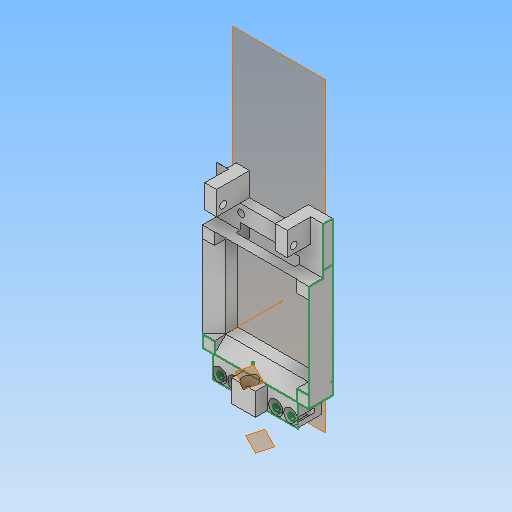
# Autodesk Inventor part: 09_Opentrons_Autofocus_LED_Module
Saved by Autodesk Inventor 2019.4 (Build 234330000, 330)
## iProperties
Created: 2020-11-27
Part Number: 09_Opentrons_Autofocus_LED_Module
Material: Generic
Document SubType Name: Modeling
Designer: diederichbenedict
Density: 1 g/cm^3
Appearance: Default
Author: diederichbenedict
Autodesk Inventor part; units mm, degrees
ref_plane "YZ Plane" through (0, 0, 0) normal (1, 0, 0) x (0, 1, 0)
ref_plane "XZ Plane" through (0, 0, 0) normal (0, 1, 0) x (-1, 0, 0)
ref_plane "XY Plane" through (0, 0, 0) normal (0, 0, 1) x (1, 0, 0)
ref_plane "Work Plane1" through (0, 0, 0) normal (0, 0, 1) x (1, 0, 0)
sketch "Sketch1" plane through (0, 0, 0) normal (0, 0, 1) x (1, 0, 0)
  circle A0 centre (8.8475, 49.7489) radius 1.45 construction
  circle A1 centre (9.593, -3.6603) radius 1.45 construction
  circle A2 centre (-7.7223, -3.6603) radius 1.45 construction
  circle A3 centre (-14.1116, -11.6603) radius 1.45 construction
  circle A4 centre (-7.7223, -11.6603) radius 1.45 construction
  circle A5 centre (9.593, -11.6603) radius 1.45 construction
  circle A6 centre (15.9823, -11.6603) radius 1.45 construction
  circle A7 centre (-6.9768, 49.7489) radius 1.45 construction
  line L0 (-17.1585, 69.3865) -> (-2.1585, 69.3865) construction
  line L1 (-2.1585, 69.3865) -> (-2.1585, 62.7008) construction
  line L2 (-2.1585, 62.7008) -> (-2.1585, 59.9787) construction
  line L3 (-2.1585, 59.9787) -> (-2.1585, 53.293) construction
  line L4 (-2.1585, 53.293) -> (-17.1585, 53.293) construction
  line L5 (-17.1585, 53.293) -> (-17.1585, -14.6603) construction
  line L6 (-17.1585, -14.6603) -> (18.8415, -14.6603) construction
  line L7 (18.8415, -14.6603) -> (18.8415, 91.3397) construction
  line L8 (-6.8647, 91.3397) -> (18.8415, 91.3397) construction
  line L9 (-6.8647, 103.3397) -> (-6.8647, 91.3397) construction
  line L10 (-17.1585, 103.3397) -> (-6.8647, 103.3397) construction
  line L11 (-17.1585, 69.3865) -> (-17.1585, 103.3397) construction
  line L12 (18.4353, 34.7801) -> (-16.5647, 34.7801)
  line L13 (-16.5647, 34.7801) -> (-16.5647, -0.2199)
  line L14 (-16.5647, -0.2199) -> (18.4353, -0.2199)
  line L15 (18.4353, -0.2199) -> (18.4353, 34.7801)
  line L16 (18.4353, 34.7801) -> (-16.5647, -0.2199) construction
  line L17 (-16.5647, 34.7801) -> (18.4353, -0.2199) construction
  line L18 (23.4353, -5.2199) -> (-21.5647, -5.2199)
  line L19 (-21.5647, -5.2199) -> (-21.5647, 39.7801)
  line L20 (-21.5647, 39.7801) -> (23.4353, 39.7801)
  line L21 (23.4353, 39.7801) -> (23.4353, -5.2199)
  line L22 (23.4353, -5.2199) -> (-21.5647, 39.7801) construction
  line L23 (-21.5647, -5.2199) -> (23.4353, 39.7801) construction
  line L24 (-17.1585, -14.6603) -> (18.8415, -14.6603)
  line L25 (18.8415, -14.6603) -> (18.8415, -5.2199)
  line L26 (18.8415, -5.2199) -> (-17.1585, -5.2199)
  line L27 (-17.1585, -5.2199) -> (-17.1585, -14.6603)
  circle A8 centre (-14.1116, -11.6603) radius 1.45
  circle A9 centre (-7.7223, -11.6603) radius 1.45
  circle A10 centre (9.593, -11.6603) radius 1.45
  circle A11 centre (15.9823, -11.6603) radius 1.45
  line L28 (15.9353, 32.2801) -> (15.9353, 2.2801) projected
  line L29 (15.9353, 2.2801) -> (-14.0647, 2.2801) projected
  line L30 (-14.0647, 2.2801) -> (-14.0647, 32.2801) projected
  line L31 (-14.0647, 32.2801) -> (15.9353, 32.2801) projected
  point P0 (0, 0)
  point P1 (0.9353, 17.2801)
  dimension "d0" = 35
  dimension "d1" = 35
  dimension "d2" = 45
  dimension "d3" = 45
  constraints: 32 end point, 6 parallel, 4 centre point, 4 coincident, 4 concentric, 4 midpoint, 3 horizontal, 3 perpendicular, 2 point on line
  measures "d0" distance of L14.end L13.end
  measures "d1" distance of L13.end L12.end
  measures "d2" distance of L19.end L20.end
  measures "d3" distance of L18.end L19.end
extrude "Extrusion1" add sketch "Sketch1" along normal blind 10 contours L18 L19 L20 L21 | L25 L24 L27 L18
sketch "Sketch2" plane through (-16.5647, 34.7801, 0) normal (0, -1, 0) x (1, 0, 0)
  line L0 (0, 0) -> (0, 10) projected
  line L1 (35, 0) -> (0, 0) projected
  line L2 (35, 0) -> (35, 10) projected
  line L3 (0, 10) -> (35, 10) projected
  line L4 (0, 0) -> (0, 10) projected
  line L5 (5, 0) -> (-5, 10)
  line L6 (5, 0) -> (19.1421, 0) construction
  line L7 (-5, 10) -> (5, 10)
  line L8 (40, 10) -> (-5, 10) projected
  line L9 (5, 0) -> (5, 10)
  line L10 (-5, 0) -> (-5, 10) projected
  line L11 (12.5, -7.6051) -> (12.5, -58.2325)
  line L12 (40, 10) -> (30, 0)
  line L13 (40, 0) -> (-5, 0) projected
  line L14 (40, 10) -> (54.1421, 10) construction
  line L15 (30, 0) -> (40, 10)
  line L16 (30, 0) -> (30, 10)
  line L17 (30, 0) -> (40, 0) construction
  line L18 (30, 10) -> (40, 10)
  point P0 (16.5647, 0)
  dimension "d6" = 135
  dimension "d7" = 10
  dimension "d9" = 45
  dimension "d10" = 0
  dimension "d11" = 135
  dimension "d12" = 90
  constraints: 22 end point, 3 equal length, 3 horizontal, 2 point on line, 1 collinear, 1 perpendicular, 1 vertical, 4 other
  measures "d6" angle of L6 L5
  measures "d7" distance of L7.end L5.start
  measures "d9" angle of L7 L5
  measures "d10" distance from line of L10 L5.end
  measures "d11" angle of L12 L14
  measures "d12" angle of L17 L16
extrude "Extrusion2" cut sketch "Sketch2" along normal up to surface (35 mm away) contours L5 L7 L0 | L0 L3 L9 L5 | L9 L3 L16 L1 | L16 L3 L2 L12 | L2 L8 L12
sketch "Sketch3" plane through (0, 0, 10) normal (0, 0, 1) x (1, 0, 0)
  line L0 (23.4353, -0.2199) -> (-21.5647, -0.2199) projected
  line L1 (-21.5647, -0.2199) -> (-21.5647, -5.2199) projected
  line L2 (-21.5647, -5.2199) -> (-17.1585, -5.2199) projected
  line L3 (-17.1585, -5.2199) -> (-17.1585, -14.6603) projected
  line L4 (-17.1585, -14.6603) -> (18.8415, -14.6603) projected
  line L5 (18.8415, -14.6603) -> (18.8415, -5.2199) projected
  line L6 (18.8415, -5.2199) -> (23.4353, -5.2199) projected
  line L7 (23.4353, -5.2199) -> (23.4353, -0.2199) projected
  circle A0 centre (15.9823, -11.6603) radius 1.45 projected
  circle A1 centre (9.593, -11.6603) radius 1.45 projected
  circle A2 centre (-7.7223, -11.6603) radius 1.45 projected
  circle A3 centre (-14.1116, -11.6603) radius 1.45 projected
  circle A4 centre (0.9353, 17.3993) radius 10.125 projected
  point P0 (0, 0)
ref_plane "Work Plane2" through (0.9353, 17.3993, 8.4308) normal (0, 0, 1) x (1, 0, 0)
pattern_circular "Circular Pattern1" count 2 over 90 about axis through (0.9353, 17.3993, 10) along (0, 0, 1) of "Extrusion2"
sketch "Sketch4" plane through (0, 0, 10) normal (0, 0, 1) x (1, 0, 0)
  line L0 (-16.4454, -5.1007) -> (-16.4454, -0.2199) projected
  line L1 (-16.4454, -0.2199) -> (-21.5647, -0.2199) projected
  line L2 (-21.5647, -0.2199) -> (-21.5647, -5.2199) projected
  line L3 (-21.5647, -5.2199) -> (-17.1585, -5.2199) projected
  line L4 (-17.1585, -5.2199) -> (-17.1585, -14.6603) projected
  line L5 (-17.1585, -14.6603) -> (18.8415, -14.6603) projected
  line L6 (18.8415, -14.6603) -> (18.8415, -5.2199) projected
  line L7 (18.8415, -5.2199) -> (23.4353, -5.2199) projected
  line L8 (23.4353, -5.2199) -> (23.4353, -0.2199) projected
  line L9 (23.4353, -0.2199) -> (18.5546, -0.2199) projected
  line L10 (18.5546, -0.2199) -> (18.5546, -5.1007) projected
  line L11 (18.5546, -5.1007) -> (-16.4454, -5.1007) projected
  circle A0 centre (15.9823, -11.6603) radius 1.45 projected
  circle A1 centre (9.593, -11.6603) radius 1.45 projected
  circle A2 centre (-7.7223, -11.6603) radius 1.45 projected
  circle A3 centre (-14.1116, -11.6603) radius 1.45 projected
  point P0 (0, 0)
hole "Hole1" at (-14.1116, -11.6603, 10) at (-7.7223, -11.6603, 10) at (9.593, -11.6603, 10) at (15.9823, -11.6603, 10) direction (0, 0, -1) diameter 2.9 end through all counterbore diameter 6 counterbore depth 7
sketch "Sketch5" plane through (0, 0, 10) normal (0, 0, 1) x (1, 0, 0)
  line L0 (-2.5647, -10.9312) -> (-2.5647, -13.1962)
  line L1 (4.4353, -10.9312) -> (4.4353, -13.1962)
  line L2 (-7.7223, -14.6603) -> (9.593, -14.6603) projected
  line L3 (18.5546, -5.1007) -> (-16.4454, -5.1007) projected
  line L4 (5.9353, -5.1007) -> (-4.0647, -5.1007)
  line L5 (-4.0647, -5.1007) -> (-4.0647, -14.6603)
  line L6 (-4.0647, -14.6603) -> (5.9353, -14.6603)
  line L7 (5.9353, -14.6603) -> (5.9353, -5.1007)
  line L8 (5.9353, -5.1007) -> (-4.0647, -14.6603) construction
  line L9 (-4.0647, -5.1007) -> (5.9353, -14.6603) construction
  point P0 (0, 0)
  point P1 (0.9353, -9.8805)
  dimension "d25" = 0
  dimension "d26" = 10
  constraints: 16 end point, 2 midpoint, 2 parallel, 2 vertical, 1 horizontal, 1 perpendicular, 1 point on line, 4 other
  measures "d25" distance between parallel lines of L3 L4
  measures "d26" distance between parallel lines of L7 L5
extrude "Extrusion3" add sketch "Sketch5" along normal blind 5
ref_plane "Work Plane3" through (3.4683, -3.8016, 13.7177) normal (0, 0.9848078, 0.173648) x (0.426172, 0.1570893, -0.8908986)
sketch "Sketch6" plane through (3.4683, -3.8016, 13.7177) normal (0, 0.9848078, 0.173648) x (0.426172, 0.1570893, -0.8908986)
  circle A0 centre (0, 2.8) radius 3 projected
  circle A1 centre (0, 2.8) radius 3
  point P0 (11.3402, 9.1762)
  dimension "d29" = 6
  constraints: 1 centre point, 1 coincident
  measures "d29" diameter of A1
extrude "Extrusion4" cut sketch "Sketch6" against normal through all
ref_plane "Work Plane4" through (3.4683, -29.6528, 9.1595) normal (0, 0.9848078, 0.173648) x (0.426172, 0.1570893, -0.8908986)
sketch "Sketch7" plane through (3.4683, -29.6528, 9.1595) normal (0, 0.9848078, 0.173648) x (0.426172, 0.1570893, -0.8908986)
  circle A0 centre (0, 2.8) radius 3.5 projected
  circle A1 centre (0, 2.8) radius 4
  point P0 (11.3402, 9.1762)
  dimension "d33" = 8
  constraints: 1 centre point, 1 coincident
  measures "d33" diameter of A1
ref_plane "Work Plane5" through (-3.7225, -12.4362, 6.5391) normal (0, -0.9848078, -0.173648) x (0.9046422, -0.0740039, 0.4196975)
extrude "Extrusion5" cut sketch "Sketch7" along normal up to surface (16.5 mm away) contours A0 | A1
sketch "Sketch8" plane through (-21.5647, 39.7801, 0) normal (0, 1, 0) x (1, 0, 0)
  line L0 (5.1193, -10) -> (5.1193, -9.8807) projected
  line L1 (5.1193, -9.8807) -> (40.1193, -9.8807) projected
  line L2 (40.1193, -9.8807) -> (40.1193, -10) projected
  line L3 (45, -10) -> (40.1193, -10) projected
  line L4 (45, 0) -> (45, -10) projected
  line L5 (45, 0) -> (0, 0) projected
  line L6 (0, 0) -> (0, -10) projected
  line L7 (5.1193, -10) -> (0, -10) projected
  line L8 (30.575, -5.7143) -> (27, -5.7143) projected
  line L9 (30.575, -5.7143) -> (30.575, -4.7143) projected
  line L10 (27, -4.7143) -> (30.575, -4.7143) projected
  line L11 (18, -4.7143) -> (27, -4.7143) projected
  line L12 (14.425, -4.7143) -> (18, -4.7143) projected
  line L13 (14.425, -5.7143) -> (14.425, -4.7143) projected
  line L14 (18, -5.7143) -> (14.425, -5.7143) projected
  line L15 (27, -5.7143) -> (18, -5.7143) projected
  line L16 (5, 0) -> (40, 0) projected
  line L17 (35, -5.7143) -> (10, -5.7143)
  line L18 (10, -5.7143) -> (10, 0)
  line L19 (10, 0) -> (35, 0)
  line L20 (35, 0) -> (35, -5.7143)
  point P0 (21.5647, 0)
  dimension "d36" = 10
  dimension "d37" = 10
  constraints: 8 end point, 2 parallel, 1 horizontal, 1 perpendicular, 1 point on line
  measures "d36" distance between parallel lines of L20 L4
  measures "d37" distance between parallel lines of L6 L18
extrude "Extrusion6" cut sketch "Sketch8" against normal up to surface (5 mm away) contours L5 L20 L17 L9 L10 L11 L12 L13 L18 | L13 L12 L11 L10 L9 L8 L15 L14
sketch "Sketch9" plane through (0, 0, 0) normal (0, 0, -1) x (-1, 0, 0)
  line L0 (-13.4353, 34.7801) -> (-13.4353, 39.7801) projected
  line L1 (-23.4353, 39.7801) -> (-13.4353, 39.7801) projected
  line L2 (-23.4353, -5.2199) -> (-23.4353, 39.7801) projected
  line L3 (-18.8415, -5.2199) -> (-23.4353, -5.2199) projected
  line L4 (-18.8415, -14.6603) -> (-18.8415, -5.2199) projected
  line L5 (17.1585, -14.6603) -> (-18.8415, -14.6603) projected
  line L6 (17.1585, -5.2199) -> (17.1585, -14.6603) projected
  line L7 (21.5647, -5.2199) -> (17.1585, -5.2199) projected
  line L8 (21.5647, 39.7801) -> (21.5647, -5.2199) projected
  line L9 (11.5647, 39.7801) -> (21.5647, 39.7801) projected
  line L10 (11.5647, 39.7801) -> (11.5647, 34.7801) projected
  line L11 (11.5647, 34.7801) -> (16.5647, 34.7801) projected
  line L12 (16.5647, 34.7801) -> (16.5647, -0.2199) projected
  line L13 (16.5647, -0.2199) -> (-18.4353, -0.2199) projected
  line L14 (-18.4353, -0.2199) -> (-18.4353, 4.8993) projected
  line L15 (-18.4353, 4.8993) -> (-18.5546, 4.8993) projected
  line L16 (-18.5546, 4.8993) -> (-18.5546, 29.8993) projected
  line L17 (-18.5546, 29.8993) -> (-18.4353, 29.8993) projected
  line L18 (-18.4353, 29.8993) -> (-18.4353, 34.7801) projected
  line L19 (-18.4353, 34.7801) -> (-13.4353, 34.7801) projected
  circle A0 centre (14.1116, -11.6603) radius 1.45 projected
  circle A1 centre (7.7223, -11.6603) radius 1.45 projected
  circle A2 centre (-9.593, -11.6603) radius 1.45 projected
  circle A3 centre (-15.9823, -11.6603) radius 1.45 projected
  line L20 (-8.9353, 55.6182) -> (7.0647, 55.6182) projected
  line L21 (7.0647, 55.6182) -> (7.0647, 61.2182) projected
  line L22 (7.0647, 61.2182) -> (-8.9353, 61.2182) projected
  line L23 (-8.9353, 61.2182) -> (-8.9353, 55.6182) projected
  circle A4 centre (7.6659, 72.0993) radius 0.5 projected
  circle A5 centre (-9.7637, 72.0993) radius 0.5 projected
  line L24 (3.5647, 69.0382) -> (3.5647, 73.4382) projected
  line L25 (3.5647, 73.4382) -> (7.1397, 73.4382) projected
  arc A6 (9.1397, 71.4382) -> (7.1397, 73.4382) centre (7.1397, 71.4382) ccw projected
  line L26 (9.1397, 71.4382) -> (9.1397, 32.1382) projected
  arc A7 (7.1397, 30.1382) -> (9.1397, 32.1382) centre (7.1397, 32.1382) ccw projected
  line L27 (7.1397, 30.1382) -> (-9.0103, 30.1382) projected
  arc A8 (-11.0103, 32.1382) -> (-9.0103, 30.1382) centre (-9.0103, 32.1382) ccw projected
  line L28 (-11.0103, 32.1382) -> (-11.0103, 71.4382) projected
  arc A9 (-9.0103, 73.4382) -> (-11.0103, 71.4382) centre (-9.0103, 71.4382) ccw projected
  line L29 (-9.0103, 73.4382) -> (-5.4353, 73.4382) projected
  line L30 (-5.4353, 73.4382) -> (-5.4353, 69.0382) projected
  line L31 (-5.4353, 69.0382) -> (3.5647, 69.0382) projected
  line L32 (-23.4353, 39.7801) -> (-13.4353, 39.7801)
  line L33 (-13.4353, 39.7801) -> (-13.4353, 42.7801)
  line L34 (-13.4353, 42.7801) -> (-23.4353, 42.7801)
  line L35 (-23.4353, 42.7801) -> (-23.4353, 39.7801)
  line L36 (21.5647, 39.7801) -> (11.5647, 39.7801)
  line L37 (11.5647, 39.7801) -> (11.5647, 42.7801)
  line L38 (11.5647, 42.7801) -> (21.5647, 42.7801)
  line L39 (21.5647, 42.7801) -> (21.5647, 39.7801)
  line L40 (-23.4353, 42.7801) -> (21.5647, 42.7801)
  line L41 (21.5647, 42.7801) -> (21.5647, 49.7801)
  line L42 (21.5647, 49.7801) -> (-23.4353, 49.7801)
  line L43 (-23.4353, 49.7801) -> (-23.4353, 42.7801)
  line L44 (21.5647, 49.7801) -> (11.5647, 49.7801)
  line L45 (11.5647, 49.7801) -> (11.5647, 59.7801)
  line L46 (11.5647, 59.7801) -> (21.5647, 59.7801)
  line L47 (21.5647, 59.7801) -> (21.5647, 49.7801)
  line L48 (-23.4353, 49.7801) -> (-13.4353, 49.7801)
  line L49 (-13.4353, 49.7801) -> (-13.4353, 59.7801)
  line L50 (-13.4353, 59.7801) -> (-23.4353, 59.7801)
  line L51 (-23.4353, 59.7801) -> (-23.4353, 49.7801)
  circle A10 centre (11.1397, 46.2801) radius 1.45
  circle A11 centre (-13.0103, 46.2801) radius 1.45
  point P0 (0, 0)
  dimension "d40" = 3
  dimension "d42" = 7
  dimension "d45" = 10
  dimension "d46" = 10
  dimension "d47" = 10
  dimension "d48" = 10
  dimension "d54" = 2.9
  dimension "d55" = 2.9
  dimension "d56" = 2
  dimension "d57" = 2
  constraints: 40 end point, 10 parallel, 5 horizontal, 5 perpendicular, 2 centre point, 2 point on line
  measures "d40" distance of L33.end L32.end
  measures "d42" distance of L41.end L40.end
  measures "d45" distance of L45.end L46.end
  measures "d46" distance of L44.end L45.end
  measures "d47" distance of L50.end L49.end
  measures "d48" distance of L49.end L48.end
  measures "d54" diameter of A10
  measures "d55" diameter of A11
  measures "d56" distance from line of A10.centre L26
  measures "d57" distance from line of L28 A11.centre
extrude "Extrusion7" add sketch "Sketch9" against normal blind 4 contours L1 L35 L34 L33 | L34 L43 L42 L28 L40 | L28 L42 L26 L40 | L51 L50 L49 L42 | L26 L42 L41 L38 L40 | L38 L39 L9 L37 | L45 L46 L47 L42
sketch "Sketch10" plane through (23.4353, -5.2199, 10) normal (1, 0, 0) x (0, 0, -1)
  line L0 (10, 48) -> (6, 48) projected
  line L1 (10, 0) -> (10, 65) projected
  line L2 (6, 45) -> (6, 65) projected
  line L3 (6, 45) -> (0, 45) projected
  line L4 (0, 40) -> (0, 45) projected
  line L5 (0, 5) -> (0, 40) projected
  line L6 (0, 0) -> (0, 5) projected
  line L7 (10, 0) -> (0, 0) projected
  line L8 (10, 65) -> (6, 65) projected
  point P0 (10, 5.2199)
sketch "Sketch11" plane through (13.4353, -5.2199, 10) normal (1, 0, 0) x (0, 0, -1)
  line L0 (10, 0) -> (10, 65) projected
  line L1 (10, 65) -> (6, 65) projected
  line L2 (6, 45) -> (6, 65) projected
  line L3 (6, 45) -> (0, 45) projected
  line L4 (0, 40) -> (0, 45) projected
  line L5 (0, 5) -> (0, 40) projected
  line L6 (0, 0) -> (0, 5) projected
  line L7 (10, 0) -> (0, 0) projected
  line L8 (4.1927, 55.6081) -> (-4.7691, 57.1883) projected
  circle A0 centre (-1.2507, 58.0402) radius 1.45
  line L9 (6, 65) -> (-4, 65)
  line L10 (-4, 65) -> (-4, 55)
  line L11 (-4, 55) -> (6, 55)
  line L12 (6, 55) -> (6, 65)
  point P0 (10, 5.2199)
  dimension "d49" = 2.9
  dimension "d50" = 10
  dimension "d51" = 10
  constraints: 8 end point, 2 parallel, 1 centre point, 1 horizontal, 1 perpendicular, 1 tangent
  measures "d49" diameter of A0
  measures "d50" distance of L11.end L10.end
  measures "d51" distance of L10.end L9.end
extrude "Extrusion8" add sketch "Sketch11" along normal blind 5 contours L2 L11 L10 L9
sketch "Sketch12" plane through (-11.5647, 49.7801, 0) normal (1, 0, 0) x (0, 0, -1)
  circle A0 centre (-11.2507, 3.0402) radius 1.45 projected
  line L0 (-4, 10) -> (-4, 0) projected
  line L1 (-4, 10) -> (-14, 10) projected
  line L2 (-14, 10) -> (-14, 0) projected
  line L3 (-14, 0) -> (-4, 0) projected
  point P0 (0, -49.7801)
extrude "Extrusion9" add sketch "Sketch12" against normal blind 5
sketch "Sketch13" plane through (-21.5647, -5.2199, 0) normal (-1, 0, 0) x (0, 0, 1)
  circle A0 centre (-7.5, 66.5596) radius 11 projected
  circle A1 centre (-7.5, 66.5596) radius 11.5
  point P0 (0, 5.2199)
  dimension "d60" = 0.5
  constraints: 1 centre point
  measures "d60" radial gap between concentric circles of A0 A1
ref_plane "Work Plane6" through (-17.1585, -14.6603, -22) normal (-1, 0, 0) x (0, 0, 1)
extrude "Extrusion10" cut sketch "Sketch13" against normal up to surface (4.4061 mm away) contours A0 | A1
body "Solid1"
